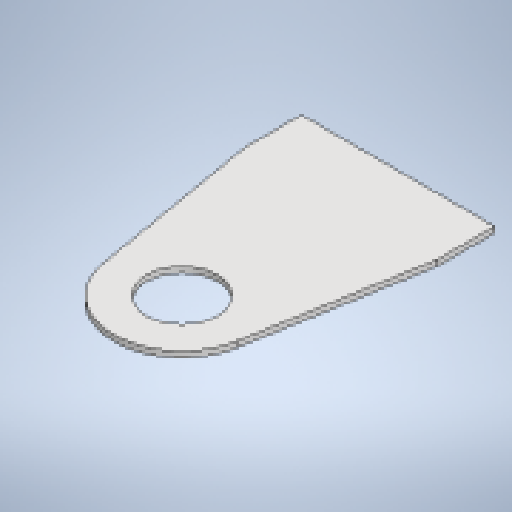
# Autodesk Inventor part: NVPH-301 back side
Saved by Autodesk Inventor 2025.1 (Build 291241020, 241B)
## iProperties
Created: 2024-12-03
Part Number: NVPH-301 back side
Material: Generic
Document SubType Name: Sheet Metal
Designer: user
Density: 1 g/cm^3
Sheet Metal Rule: Default
Appearance: Default
Flat Pattern Width: 50 cm
Flat Pattern Length: 34 cm
Flat Pattern Area: 1700 cm^2
Sheet Metal Width: 500.000 mm
Sheet Metal Length: 340.000 mm
Sheet Metal Area: 170000.000 mm^2
Author: user
Autodesk Inventor part; units mm, degrees
ref_plane "YZ Plane" through (0, 0, 0) normal (1, 0, 0) x (0, 1, 0)
ref_plane "XZ Plane" through (0, 0, 0) normal (0, 1, 0) x (-1, 0, 0)
ref_plane "XY Plane" through (0, 0, 0) normal (0, 0, 1) x (1, 0, 0)
sketch "Sketch1" plane through (0, 0, 0) normal (0, 0, 1) x (1, 0, 0)
  line L0 (0, 0) -> (0, 500)
  line L1 (-170, 500) -> (170, 500)
  circle A0 centre (0, 120) radius 62.5
  circle A1 centre (0, 120) radius 120
  line L2 (-170, 500) -> (-170, 400)
  line L3 (-170, 400) -> (-118.2583, 99.6289)
  line L4 (170, 500) -> (170, 400)
  line L5 (170, 400) -> (118.2583, 99.6289)
  dimension "d0" = 500
  dimension "d1" = 340
  dimension "d2" = 125
  dimension "d4" = 100
  dimension "d16" = 19.548
  dimension "d17" = 240
  measures "d0" distance of L0.end L0.start
  measures "d1" distance of L1.start L1.end
  measures "d2" diameter of A0
  measures "d4" distance of L1.start L2.end
  measures "d16" angle of L5 L3
  measures "d17" diameter of A1
extrude "Plate1" add sketch "Sketch1" along normal blind 10 contours A1 L0 A0 | L0 A0 A1 | L3 L2 L1 L0 A1 | A1 L0 L1 L4 L5
sketch "Sketch2" plane through (-170, 491.3397, 5) normal (0, 0.8660254, -0.5) x (-1, 0, 0)
  line L0 (-340, 0) -> (0, 0)
  line L1 (0, 0) -> (0, 40)
  line L2 (0, 40) -> (-340, 40)
  line L3 (-340, 40) -> (-340, 0)
  constraints: 6 end point, 1 horizontal, 1 perpendicular, 1 vertical
equation "\"d2\" = back_steel_circle_проходной_диаметр"
equation "\"d5\" = Thickness"
equation "\"BendReliefDepth\" = 0.5 * Thickness"
equation "\"back_steel_circle_проходной_диаметр\" = 125"
equation "\"Thickness\" = 10"
body "Solid1"
